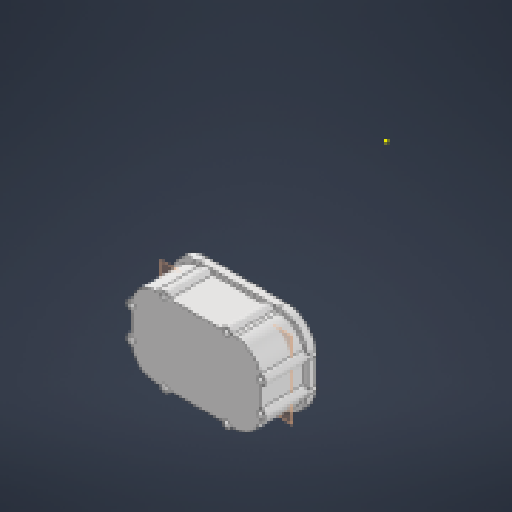
# Autodesk Inventor part: front_main_body
Saved by Autodesk Inventor 2024 (Build 280153000, 153)
## iProperties
Created: 2026-08-19
Part Number: front_main_body
Material: Generic
Document SubType Name: Modeling
Designer: schar
Density: 1 g/cm^3
Appearance: Default
Author: schar
Autodesk Inventor part; units mm, degrees
ref_plane "YZ Plane" through (0, 0, 0) normal (1, 0, 0) x (0, 1, 0)
ref_plane "XZ Plane" through (0, 0, 0) normal (0, 1, 0) x (-1, 0, 0)
ref_plane "XY Plane" through (0, 0, 0) normal (0, 0, 1) x (1, 0, 0)
ref_plane "Work Plane1" through (0, 0, 0) normal (0, 0, 1) x (1, 0, 0)
sketch "Sketch1" plane through (0, 0, 0) normal (0, 0, 1) x (1, 0, 0)
  circle A0 centre (-97.4, -116.425) radius 0.5 projected
  circle A1 centre (-82.2, -105.3) radius 1.6 projected
  circle A2 centre (-57.8, -105.3) radius 1.6 projected
  circle A3 centre (-49.4, -113.69) radius 0.5 projected
  circle A4 centre (-49.4, -116.23) radius 0.5 projected
  circle A5 centre (-97.4, -118.965) radius 0.5 projected
  circle A6 centre (-49.4, -118.77) radius 0.5 projected
  circle A7 centre (-49.4, -121.31) radius 0.5 projected
  circle A8 centre (-82.2, -129.7) radius 1.6 projected
  circle A9 centre (-57.8, -129.7) radius 1.6 projected
  line L0 (-100, -110) -> (-100, -125) projected
  arc A10 (-100, -125) -> (-90, -135) centre (-90, -125) ccw projected
  line L1 (-90, -135) -> (-50, -135) projected
  arc A11 (-50, -135) -> (-40, -125) centre (-50, -125) ccw projected
  line L2 (-40, -125) -> (-40, -110) projected
  arc A12 (-40, -110) -> (-50, -100) centre (-50, -110) ccw projected
  line L3 (-50, -100) -> (-90, -100) projected
  arc A13 (-90, -100) -> (-100, -110) centre (-90, -110) ccw projected
  circle A14 centre (-82.2, -105.3) radius 1.6
  circle A15 centre (-82.2, -105.3) radius 2.5
  circle A16 centre (-57.8, -105.3) radius 1.6
  circle A17 centre (-57.8, -105.3) radius 2.5
  circle A18 centre (-57.8, -129.7) radius 1.6
  circle A19 centre (-57.8, -129.7) radius 2.5
  circle A20 centre (-82.2, -129.7) radius 1.6
  circle A21 centre (-82.2, -129.7) radius 2.5
  line L4 (-90, -97.5) -> (-50, -97.5)
  arc A22 (-37.5, -110) -> (-50, -97.5) centre (-50, -110) ccw
  line L5 (-37.5, -110) -> (-37.5, -125)
  arc A23 (-50, -137.5) -> (-37.5, -125) centre (-50, -125) ccw
  line L6 (-50, -137.5) -> (-90, -137.5)
  arc A24 (-102.5, -125) -> (-90, -137.5) centre (-90, -125) ccw
  line L7 (-102.5, -125) -> (-102.5, -110)
  arc A25 (-90, -97.5) -> (-102.5, -110) centre (-90, -110) ccw
  point P0 (0, 0)
  dimension "d0" = 5
  dimension "d1" = 5
  dimension "d2" = 5
  dimension "d3" = 5
  dimension "d4" = 2.5
  constraints: 12 centre point, 8 coincident, 8 end point, 8 point on circle, 4 concentric, 7 other
  measures "d0" diameter of A15
  measures "d1" diameter of A17
  measures "d2" diameter of A19
  measures "d3" diameter of A21
  measures "d4" distance between parallel lines of L3 L4
extrude "Extrusion1" add sketch "Sketch1" along normal blind 13 contours A15 | A17 | A19 | A21 | L4 A22 L5 A23 L6 A24 L7 A25
sketch "Sketch2" plane through (0, 0, 13) normal (0, 0, 1) x (1, 0, 0)
  line L0 (-50, -97.5) -> (-90, -97.5) projected
  arc A0 (-37.5, -110) -> (-50, -97.5) centre (-50, -110) ccw projected
  line L1 (-37.5, -125) -> (-37.5, -110) projected
  arc A1 (-50, -137.5) -> (-37.5, -125) centre (-50, -125) ccw projected
  line L2 (-90, -137.5) -> (-50, -137.5) projected
  arc A2 (-102.5, -125) -> (-90, -137.5) centre (-90, -125) ccw projected
  line L3 (-102.5, -110) -> (-102.5, -125) projected
  arc A3 (-90, -97.5) -> (-102.5, -110) centre (-90, -110) ccw projected
  point P0 (0, 0)
extrude "Extrusion2" add sketch "Sketch2" along normal blind 2.5
sketch "Sketch3" plane through (0, 0, 0) normal (0, 0, -1) x (-1, 0, 0)
  line L0 (90, -137.5) -> (50, -137.5) projected
  arc A0 (90, -137.5) -> (102.5, -125) centre (90, -125) ccw projected
  line L1 (102.5, -110) -> (102.5, -125) projected
  arc A1 (102.5, -110) -> (90, -97.5) centre (90, -110) ccw projected
  line L2 (50, -97.5) -> (90, -97.5) projected
  arc A2 (50, -97.5) -> (37.5, -110) centre (50, -110) ccw projected
  line L3 (37.5, -125) -> (37.5, -110) projected
  arc A3 (37.5, -125) -> (50, -137.5) centre (50, -125) ccw projected
  arc A4 (100, -110) -> (90, -100) centre (90, -110) ccw projected
  line L4 (100, -125) -> (100, -110) projected
  arc A5 (90, -135) -> (100, -125) centre (90, -125) ccw projected
  line L5 (50, -135) -> (90, -135) projected
  arc A6 (40, -125) -> (50, -135) centre (50, -125) ccw projected
  line L6 (40, -110) -> (40, -125) projected
  arc A7 (50, -100) -> (40, -110) centre (50, -110) ccw projected
  line L7 (90, -100) -> (50, -100) projected
  point P0 (0, 0)
extrude "Extrusion3" add sketch "Sketch3" along normal blind 10
sketch "Sketch4" plane through (-82.2, -129.7, 13) normal (0, 0, -1) x (-1, 0, 0)
  circle A0 centre (0, 0) radius 1.6 projected
  circle A1 centre (0, 24.4) radius 1.6 projected
  circle A2 centre (-24.4, 24.4) radius 1.6 projected
  circle A3 centre (-24.4, 0) radius 1.6 projected
  circle A4 centre (0, 0) radius 1.5
  circle A5 centre (-24.4, 0) radius 1.5
  circle A6 centre (-24.4, 24.4) radius 1.5
  circle A7 centre (0, 24.4) radius 1.5
  point P0 (-82.2, 129.7)
  dimension "d11" = 3
  dimension "d12" = 3
  dimension "d13" = 3
  dimension "d14" = 3
  constraints: 4 centre point, 4 coincident
  measures "d11" diameter of A4
  measures "d12" diameter of A5
  measures "d13" diameter of A6
  measures "d14" diameter of A7
extrude "Extrusion4" add sketch "Sketch4" along normal up to surface (13 mm away)
sketch "Sketch5" plane through (0, 0, -10) normal (0, 0, -1) x (-1, 0, 0)
  line L0 (100, -125) -> (100, -110) projected
  arc A0 (100, -110) -> (90, -100) centre (90, -110) ccw projected
  line L1 (50, -100) -> (90, -100) projected
  arc A1 (50, -100) -> (40, -110) centre (50, -110) ccw projected
  line L2 (40, -125) -> (40, -110) projected
  arc A2 (40, -125) -> (50, -135) centre (50, -125) ccw projected
  line L3 (90, -135) -> (50, -135) projected
  arc A3 (90, -135) -> (100, -125) centre (90, -125) ccw projected
  circle A4 centre (57.8, -129.7) radius 1.6 projected
  circle A5 centre (82.2, -129.7) radius 1.6 projected
  circle A6 centre (49.4, -121.31) radius 0.5 projected
  circle A7 centre (49.4, -118.77) radius 0.5 projected
  circle A8 centre (97.4, -118.965) radius 0.5 projected
  circle A9 centre (49.4, -116.23) radius 0.5 projected
  circle A10 centre (49.4, -113.69) radius 0.5 projected
  circle A11 centre (57.8, -105.3) radius 1.6 projected
  circle A12 centre (82.2, -105.3) radius 1.6 projected
  circle A13 centre (97.4, -116.425) radius 0.5 projected
  arc A14 (100.2, -110) -> (90, -99.8) centre (90, -110) ccw
  line L4 (100.2, -110) -> (100.2, -125)
  arc A15 (90, -135.2) -> (100.2, -125) centre (90, -125) ccw
  line L5 (90, -135.2) -> (50, -135.2)
  arc A16 (39.8, -125) -> (50, -135.2) centre (50, -125) ccw
  line L6 (39.8, -125) -> (39.8, -110)
  arc A17 (50, -99.8) -> (39.8, -110) centre (50, -110) ccw
  line L7 (50, -99.8) -> (90, -99.8)
  point P0 (0, 0)
  dimension "d17" = 0.2
  constraints: 8 end point, 8 point on circle, 4 centre point, 7 other
  measures "d17" distance between parallel lines of L1 L7
extrude "Extrusion5" cut sketch "Sketch5" against normal up to surface (23 mm away) contours L4 A15 L5 A16 L6 A17 L7 A14
sketch "Sketch6" plane through (0, 0, -10) normal (0, 0, -1) x (-1, 0, 0)
  point P0 (0, 0)
sketch "Sketch8" plane through (0, 0, -10) normal (0, 0, -1) x (-1, 0, 0)
  line L0 (90, -99.8) -> (50, -99.8) projected
  line L1 (50, -99.8) -> (54.5, -99.8)
  line L2 (54.5, -99.8) -> (54.5, -97.8)
  circle A0 centre (54.5, -97.8) radius 1.5
  circle A1 centre (54.5, -97.8) radius 2.5
  line L3 (50, -99.8) -> (90, -99.8)
  line L4 (90, -135.2) -> (50, -135.2) projected
  line L5 (50, -135.2) -> (90, -135.2)
  line L6 (90, -135.2) -> (70, -135.2)
  line L7 (50, -99.8) -> (90, -99.8) projected
  line L8 (70, -99.8) -> (70, -135.2)
  circle A2 centre (85.5, -97.8) radius 1.5
  circle A3 centre (85.5, -97.8) radius 2.5
  line L9 (70, -117.5) -> (100.2, -117.5)
  line L10 (100.2, -110) -> (100.2, -125) projected
  circle A4 centre (54.5, -137.2) radius 1.5
  circle A5 centre (54.5, -137.2) radius 2.5
  circle A6 centre (85.5, -137.2) radius 2.5
  circle A7 centre (85.5, -137.2) radius 1.5
  point P0 (0, 0)
  point P1 (53, -135.2)
  point P2 (56, -135.2)
  point P3 (84, -135.2)
  point P4 (87, -135.2)
  point P5 (87, -99.8)
  point P6 (84, -99.8)
  point P7 (56, -99.8)
  point P8 (53, -99.8)
  dimension "d37" = 4.5
  dimension "d38" = 2
  dimension "d39" = 3
  dimension "d40" = 5
  constraints: 14 end point, 8 centre point, 6 symmetric about line, 5 coincident, 4 midpoint, 2 perpendicular, 1 collinear, 1 horizontal, 1 point on line, 6 other
  measures "d37" distance of L0.end L1.end
  measures "d38" distance of L1.end L2.end
  measures "d39" diameter of A0
  measures "d40" diameter of A1
extrude "Extrusion6" add sketch "Sketch8" against normal up to surface (25.5 mm away) contours L0 A3 | L0 A1 | A6 L4 | A5 L4 picked at (85.5603, -99.6297) picked at (55.2169, -99.5838) picked at (85.5603, -135.3703) picked at (54.5603, -135.3703)
sketch "Sketch9" plane through (0, 0, -10) normal (0, 0, -1) x (-1, 0, 0)
  arc A0 (84.0303, -137.5) -> (86.9697, -137.5) centre (85.5, -137.2) ccw projected
  circle A1 centre (85.5, -137.2) radius 1.5
  arc A2 (53.0303, -137.5) -> (55.9697, -137.5) centre (54.5, -137.2) ccw projected
  line L0 (53.0303, -137.5) -> (55.9697, -137.5) projected
  circle A3 centre (54.5, -137.2) radius 1.5
  arc A4 (55.9697, -97.5) -> (53.0303, -97.5) centre (54.5, -97.8) ccw projected
  circle A5 centre (54.5, -97.8) radius 1.5
  arc A6 (86.9697, -97.5) -> (84.0303, -97.5) centre (85.5, -97.8) ccw projected
  circle A7 centre (85.5, -97.8) radius 1.5
  point P0 (0, 0)
  point P1 (86.9697, -97.5)
  constraints: 4 coincident, 2 centre point, 6 other
extrude "Extrusion7" cut sketch "Sketch9" against normal up to surface (25.5 mm away)
sketch "Sketch10" plane through (0, 0, -10) normal (0, 0, -1) x (-1, 0, 0)
  line L0 (37.5, -125) -> (37.5, -110) projected
  circle A0 centre (37.5, -110) radius 1.5
  circle A1 centre (37.5, -125) radius 1.5
  arc A2 (90, -137.5) -> (102.5, -125) centre (90, -125) ccw projected
  circle A3 centre (102.5, -125) radius 1.5
  arc A4 (102.5, -110) -> (90, -97.5) centre (90, -110) ccw projected
  circle A5 centre (102.5, -110) radius 1.5
  circle A6 centre (102.5, -110) radius 2.5
  circle A7 centre (102.5, -125) radius 2.5
  circle A8 centre (37.5, -125) radius 2.5
  circle A9 centre (37.5, -110) radius 2.5
  point P0 (0, 0)
  dimension "d45" = 3
  dimension "d46" = 3
  dimension "d47" = 3
  dimension "d48" = 3
  dimension "d49" = 5
  dimension "d50" = 5
  dimension "d51" = 5
  dimension "d52" = 5
  constraints: 8 centre point, 5 coincident
  measures "d45" diameter of A0
  measures "d46" diameter of A1
  measures "d47" diameter of A3
  measures "d48" diameter of A5
  measures "d49" diameter of A6
  measures "d50" diameter of A7
  measures "d51" diameter of A8
  measures "d52" diameter of A9
extrude "Extrusion8" add sketch "Sketch10" against normal up to surface (25.5 mm away)
sketch "Sketch11" plane through (0, 0, -10) normal (0, 0, -1) x (-1, 0, 0)
  arc A0 (37.59, -108.5027) -> (37.5, -111.5) centre (37.5, -110) ccw projected
  circle A1 centre (37.5, -110) radius 1.5
  arc A2 (37.5, -125) -> (37.59, -126.4973) centre (50, -125) ccw projected
  circle A3 centre (37.5, -125) radius 1.5
  arc A4 (102.41, -126.4973) -> (102.5, -125) centre (90, -125) ccw projected
  circle A5 centre (102.5, -125) radius 1.5
  line L0 (102.5, -111.5) -> (102.5, -110) projected
  circle A6 centre (102.5, -110) radius 1.5
  point P0 (0, 0)
  constraints: 2 coincident, 1 centre point, 1 vertical alignment, 8 other
extrude "Extrusion9" cut sketch "Sketch11" against normal up to surface (25.5 mm away)
sketch "Sketch12" plane through (0, 0, -10) normal (0, 0, -1) x (-1, 0, 0)
  arc A0 (50, -99.8) -> (39.8384, -109.1158) centre (50, -110) ccw projected
  arc A1 (39.8, -110.9798) -> (39.8384, -109.1158) centre (37.5, -110) ccw projected
  line L0 (39.8, -124.0202) -> (39.8, -110.9798) projected
  arc A2 (39.8384, -125.8842) -> (50, -135.2) centre (50, -125) ccw projected
  arc A3 (39.8384, -125.8842) -> (39.8, -124.0202) centre (37.5, -125) ccw projected
  line L1 (90, -135.2) -> (50, -135.2) projected
  arc A4 (90, -135.2) -> (100.1616, -125.8842) centre (90, -125) ccw projected
  line L2 (100.2, -110.9798) -> (100.2, -124.0202) projected
  arc A5 (100.2, -124.0202) -> (100.1616, -125.8842) centre (102.5, -125) ccw projected
  arc A6 (100.1616, -109.1158) -> (90, -99.8) centre (90, -110) ccw projected
  arc A7 (100.1616, -109.1158) -> (100.2, -110.9798) centre (102.5, -110) ccw projected
  line L3 (50, -99.8) -> (90, -99.8) projected
  line L4 (39.8384, -109.1158) -> (39.8, -110.9798)
  line L5 (39.8, -110.9798) -> (39.8384, -109.1158)
  line L6 (39.8, -124.0202) -> (39.8384, -125.8842)
  line L7 (100.2, -124.0202) -> (100.1616, -125.8842)
  line L8 (100.1616, -109.1158) -> (100.2, -110.9798)
  point P0 (0, 0)
  constraints: 10 end point, 2 equal length
extrude "Extrusion10" cut sketch "Sketch12" against normal up to surface (23 mm away) contours A1 L4 | L8 A7 | A3 L6 | L7 A5
sketch "Sketch13" plane through (0, 0, -10) normal (0, 0, -1) x (-1, 0, 0)
  arc A0 (50, -97.5) -> (37.75, -107.5125) centre (50, -110) ccw projected
  line L0 (52.0181, -97.5) -> (50, -97.5) projected
  arc A1 (56.9819, -97.5) -> (52.0181, -97.5) centre (54.5, -97.8) ccw projected
  line L1 (83.0181, -97.5) -> (56.9819, -97.5) projected
  arc A2 (87.9819, -97.5) -> (83.0181, -97.5) centre (85.5, -97.8) ccw projected
  arc A3 (102.25, -107.5125) -> (90, -97.5) centre (90, -110) ccw projected
  line L2 (90, -97.5) -> (87.9819, -97.5) projected
  arc A4 (102.5, -112.5) -> (102.25, -107.5125) centre (102.5, -110) ccw projected
  line L3 (102.5, -122.5) -> (102.5, -112.5) projected
  arc A5 (102.25, -127.4875) -> (102.5, -122.5) centre (102.5, -125) ccw projected
  arc A6 (90, -137.5) -> (102.25, -127.4875) centre (90, -125) ccw projected
  line L4 (87.9819, -137.5) -> (90, -137.5) projected
  arc A7 (83.0181, -137.5) -> (87.9819, -137.5) centre (85.5, -137.2) ccw projected
  line L5 (56.9819, -137.5) -> (83.0181, -137.5) projected
  arc A8 (52.0181, -137.5) -> (56.9819, -137.5) centre (54.5, -137.2) ccw projected
  arc A9 (37.75, -127.4875) -> (50, -137.5) centre (50, -125) ccw projected
  line L6 (50, -137.5) -> (52.0181, -137.5) projected
  arc A10 (37.5, -122.5) -> (37.75, -127.4875) centre (37.5, -125) ccw projected
  line L7 (37.5, -112.5) -> (37.5, -122.5) projected
  arc A11 (37.75, -107.5125) -> (37.5, -112.5) centre (37.5, -110) ccw projected
  circle A12 centre (57.8, -129.7) radius 2.5 projected
  circle A13 centre (82.2, -129.7) radius 2.5 projected
  circle A14 centre (57.8, -105.3) radius 2.5 projected
  circle A15 centre (82.2, -105.3) radius 2.5 projected
  line L8 (100.2, -124.0202) -> (100.2, -110.9798) projected
  line L9 (100.2, -110.9798) -> (100.1616, -109.1158) projected
  arc A16 (100.1616, -109.1158) -> (90, -99.8) centre (90, -110) ccw projected
  line L10 (90, -99.8) -> (50, -99.8) projected
  arc A17 (50, -99.8) -> (39.8384, -109.1158) centre (50, -110) ccw projected
  line L11 (39.8384, -109.1158) -> (39.8, -110.9798) projected
  line L12 (39.8, -110.9798) -> (39.8, -124.0202) projected
  line L13 (39.8, -124.0202) -> (39.8384, -125.8842) projected
  arc A18 (39.8384, -125.8842) -> (50, -135.2) centre (50, -125) ccw projected
  line L14 (50, -135.2) -> (90, -135.2) projected
  arc A19 (90, -135.2) -> (100.1616, -125.8842) centre (90, -125) ccw projected
  line L15 (100.1616, -125.8842) -> (100.2, -124.0202) projected
  line L16 (50, -95.2968) -> (90, -95.2968)
  arc A20 (104.6611, -108.8875) -> (90, -95.2968) centre (90, -110) ccw
  line L17 (104.6611, -108.8875) -> (104.7032, -110.9334)
  line L18 (104.7032, -110.9334) -> (104.7032, -124.0666)
  line L19 (104.7032, -124.0666) -> (104.6611, -126.1125)
  arc A21 (90, -139.7032) -> (104.6611, -126.1125) centre (90, -125) ccw
  line L20 (90, -139.7032) -> (50, -139.7032)
  arc A22 (35.3389, -126.1125) -> (50, -139.7032) centre (50, -125) ccw
  line L21 (35.3389, -126.1125) -> (35.2968, -124.0666)
  line L22 (35.2968, -124.0666) -> (35.2968, -110.9334)
  line L23 (35.2968, -110.9334) -> (35.3389, -108.8875)
  arc A23 (50, -95.2968) -> (35.3389, -108.8875) centre (50, -110) ccw
  point P0 (0, 0)
  point P1 (35.2968, -111.1815)
  point P2 (35.2968, -123.8185)
  point P3 (35.3526, -126.2801)
  point P4 (104.6474, -126.2801)
  point P5 (104.7032, -123.8185)
  point P6 (104.7032, -111.1815)
  point P7 (104.6474, -108.7199)
  point P8 (35.3526, -108.7199)
  constraints: 16 end point, 8 point on circle, 4 centre point, 11 other
extrude "Extrusion11" add sketch "Sketch13" against normal blind 4 contours A0 A11 A23 L16 A20 A4 A3 L2 A2 L1 A1 L0 | A11 L7 A10 L22 | A10 A9 L6 A8 L5 A7 L4 A6 A5 A21 L20 A22 | L18 A5 L3 A4
sketch "Sketch14" plane through (0, 0, -10) normal (0, 0, -1) x (-1, 0, 0)
  line L0 (90, -135.2) -> (50, -135.2) projected
  arc A0 (39.8384, -125.8842) -> (50, -135.2) centre (50, -125) ccw projected
  circle A1 centre (57.8, -129.7) radius 2.5 projected
  circle A2 centre (82.2, -129.7) radius 2.5 projected
  circle A3 centre (57.8, -105.3) radius 2.5 projected
  circle A4 centre (82.2, -105.3) radius 2.5 projected
  line L1 (100.2, -124.0202) -> (100.2, -110.9798) projected
  line L2 (100.2, -110.9798) -> (100.1616, -109.1158) projected
  arc A5 (100.1616, -109.1158) -> (90, -99.8) centre (90, -110) ccw projected
  line L3 (90, -99.8) -> (50, -99.8) projected
  arc A6 (50, -99.8) -> (39.8384, -109.1158) centre (50, -110) ccw projected
  line L4 (39.8384, -109.1158) -> (39.8, -110.9798) projected
  line L5 (39.8, -110.9798) -> (39.8, -124.0202) projected
  line L6 (39.8, -124.0202) -> (39.8384, -125.8842) projected
  arc A7 (39.8384, -125.8842) -> (50, -135.2) centre (50, -125) ccw projected
  line L7 (50, -135.2) -> (90, -135.2) projected
  arc A8 (90, -135.2) -> (100.1616, -125.8842) centre (90, -125) ccw projected
  line L8 (100.1616, -125.8842) -> (100.2, -124.0202) projected
  line L9 (50, -97.8) -> (90, -97.8)
  arc A9 (102.1599, -109.0113) -> (90, -97.8) centre (90, -110) ccw
  line L10 (102.1599, -109.0113) -> (102.2, -110.9592)
  line L11 (102.2, -110.9592) -> (102.2, -124.0408)
  line L12 (102.2, -124.0408) -> (102.1599, -125.9887)
  arc A10 (90, -137.2) -> (102.1599, -125.9887) centre (90, -125) ccw
  line L13 (90, -137.2) -> (50, -137.2)
  arc A11 (37.8401, -125.9887) -> (50, -137.2) centre (50, -125) ccw
  line L14 (37.8401, -125.9887) -> (37.8, -124.0408)
  line L15 (37.8, -124.0408) -> (37.8, -110.9592)
  line L16 (37.8, -110.9592) -> (37.8401, -109.0113)
  arc A12 (50, -97.8) -> (37.8401, -109.0113) centre (50, -110) ccw
  line L17 (90, -97.3) -> (50, -97.3)
  arc A13 (50, -97.3) -> (37.3405, -108.986) centre (50, -110) ccw
  line L18 (37.3405, -108.986) -> (37.3, -110.954)
  line L19 (37.3, -110.954) -> (37.3, -124.046)
  line L20 (37.3, -124.046) -> (37.3405, -126.014)
  arc A14 (37.3405, -126.014) -> (50, -137.7) centre (50, -125) ccw
  line L21 (50, -137.7) -> (90, -137.7)
  arc A15 (90, -137.7) -> (102.6595, -126.014) centre (90, -125) ccw
  line L22 (102.6595, -126.014) -> (102.7, -124.046)
  line L23 (102.7, -124.046) -> (102.7, -110.954)
  line L24 (102.7, -110.954) -> (102.6595, -108.986)
  arc A16 (102.6595, -108.986) -> (90, -97.3) centre (90, -110) ccw
  line L25 (90, -98.3) -> (50, -98.3)
  arc A17 (50, -98.3) -> (38.3397, -109.0369) centre (50, -110) ccw
  line L26 (38.3397, -109.0369) -> (38.3, -110.9643)
  line L27 (38.3, -110.9643) -> (38.3, -124.0357)
  line L28 (38.3, -124.0357) -> (38.3397, -125.9631)
  arc A18 (38.3397, -125.9631) -> (50, -136.7) centre (50, -125) ccw
  line L29 (50, -136.7) -> (90, -136.7)
  arc A19 (90, -136.7) -> (101.6603, -125.9631) centre (90, -125) ccw
  line L30 (101.6603, -125.9631) -> (101.7, -124.0357)
  line L31 (101.7, -124.0357) -> (101.7, -110.9643)
  line L32 (101.7, -110.9643) -> (101.6603, -109.0369)
  arc A20 (101.6603, -109.0369) -> (90, -98.3) centre (90, -110) ccw
  point P0 (0, 0)
  dimension "d69" = 0.5
  dimension "d70" = 0.5
  constraints: 48 end point, 24 point on circle, 12 centre point, 33 other
  measures "d69" distance between parallel lines of L9 L17
  measures "d70" distance between parallel lines of L9 L25
extrude "Extrusion12" cut sketch "Sketch14" against normal blind 1.5 contours L9 A9 L10 L11 L12 A10 L13 A11 L14 L15 L16 A12 | A16 L24 L23 L22 A15 L21 A14 L20 L19 L18 A13 L17
thread "Thread1" size "M3x0.5" class "6H" standard "ANSI Metric M Profile" length 15.103
thread "Thread2" size "M3x0.5" class "6H" standard "ANSI Metric M Profile" length 15.103
thread "Thread3" size "M3x0.5" class "6H" standard "ANSI Metric M Profile" length 15.103
thread "Thread4" size "M3x0.5" class "6H" standard "ANSI Metric M Profile" length 15.103
sketch "Sketch15" plane through (0, 0, 15.5) normal (0, 0, 1) x (1, 0, 0)
  point P0 (0, 0)
ref_plane "Work Plane2" through (-56.9819, -97.5, 15.5) normal (0, -0.4226183, -0.9063078) x (-1, 0, 0)
ref_plane "Work Plane3" through (-56.9819, -100.4583, 9.1558) normal (0, -0.4226183, -0.9063078) x (-1, 0, 0)
ref_plane "Work Plane4" through (-84.0858, -137.7, 15.5) normal (0, 0.9063078, -0.4226183) x (1, 0, 0)
sketch "Sketch21" plane through (-84.0858, -137.7, 15.5) normal (0, 0.9063078, -0.4226183) x (1, 0, 0)
  line L0 (-1.4142, -3.55) -> (-1.4142, -16.2285) projected
  line L1 (29.5858, -16.2285) -> (29.5858, -3.55) projected
  line L2 (-1.4142, -9.8893) -> (29.5858, -9.8893)
  line L3 (29.5858, -9.8893) -> (29.5858, -7.3893)
  line L4 (29.5858, -7.3893) -> (-1.4142, -7.3893)
  line L5 (-1.4142, -7.3893) -> (-1.4142, -9.8893)
  line L6 (31.5858, -11.8893) -> (-3.4142, -11.8893)
  line L7 (-3.4142, -11.8893) -> (-3.4142, -5.3893)
  line L8 (-3.4142, -5.3893) -> (31.5858, -5.3893)
  line L9 (31.5858, -5.3893) -> (31.5858, -11.8893)
  point P0 (84.0858, -44.1468)
  point P1 (-1.4142, -7.3893)
  point P2 (29.5858, -9.8893)
  dimension "d103" = 2.5
  dimension "d104" = 2
  constraints: 16 end point, 4 parallel, 2 perpendicular, 1 horizontal, 1 midpoint, 1 point on line, 3 other
  measures "d103" distance of L3.end L2.end
  measures "d104" distance between parallel lines of L2 L6
extrude "Extrusion17" add sketch "Sketch21" along normal blind 30 contours L0 L6 L7 L8 | L0 L8 L1 L4 | L2 L1 L6 L0 | L1 L8 L9 L6
sketch "Sketch22" plane through (-84.0858, -137.7, 15.5) normal (0, 0.9063078, -0.4226183) x (1, 0, 0)
  line L0 (-1.4142, -9.8893) -> (-1.4142, -7.3893) projected
  line L1 (-1.4142, -7.3893) -> (29.5858, -7.3893) projected
  line L2 (29.5858, -7.3893) -> (29.5858, -9.8893) projected
  line L3 (29.5858, -9.8893) -> (-1.4142, -9.8893) projected
  point P0 (84.0858, -44.1468)
extrude "Extrusion18" cut sketch "Sketch22" along normal blind 30
sketch "Sketch23" plane through (-84.0858, -110.5108, 2.8215) normal (0, 0.9063078, -0.4226183) x (1, 0, 0)
  point P0 (84.0858, -44.1468)
sketch "Sketch24" plane through (-84.0858, -110.5108, 2.8215) normal (0, 0.9063078, -0.4226183) x (1, 0, 0)
  line L0 (31.5858, -5.3893) -> (-3.4142, -5.3893) projected
  line L1 (31.5858, -11.2308) -> (31.5858, -5.3893) projected
  line L2 (31.5858, -11.2308) -> (28.7423, -11.2308) projected
  line L3 (-3.4142, -5.3893) -> (-3.4142, -11.2308) projected
  line L4 (23.8293, -11.2308) -> (4.3423, -11.2308) projected
  line L5 (27.7121, -11.2308) -> (24.8595, -11.2308) projected
  line L6 (3.3121, -11.2308) -> (0.4595, -11.2308) projected
  line L7 (-0.5707, -11.2308) -> (-3.4142, -11.2308) projected
  ellipse E0 centre (26.2858, -12.3297) end of major axis (26.2858, -18.2452) minor radius 2.5 (27.6608, -7.3893) -> (24.9108, -7.3893) ccw projected
  ellipse E1 centre (26.2858, -12.3297) end of major axis (26.2858, -18.2452) minor radius 2.5 (24.9108, -7.3893) -> (24.0085, -9.8893) ccw projected
  ellipse E2 centre (26.2858, -12.3297) end of major axis (26.2858, -18.2452) minor radius 2.5 (24.0085, -9.8893) -> (23.8293, -11.2308) ccw projected
  ellipse E3 centre (26.2858, -12.3297) end of major axis (26.2858, -18.2452) minor radius 2.5 (28.5631, -9.8893) -> (27.6608, -7.3893) ccw projected
  ellipse E4 centre (26.2858, -12.3297) end of major axis (26.2858, -18.2452) minor radius 2.5 (28.7423, -11.2308) -> (28.5631, -9.8893) ccw projected
  ellipse E5 centre (1.8858, -12.3297) end of major axis (1.8858, -18.2452) minor radius 2.5 (4.3423, -11.2308) -> (4.1631, -9.8893) ccw projected
  ellipse E6 centre (1.8858, -12.3297) end of major axis (1.8858, -18.2452) minor radius 2.5 (4.1631, -9.8893) -> (3.2608, -7.3893) ccw projected
  ellipse E7 centre (1.8858, -12.3297) end of major axis (1.8858, -18.2452) minor radius 2.5 (3.2608, -7.3893) -> (0.5108, -7.3893) ccw projected
  ellipse E8 centre (1.8858, -12.3297) end of major axis (1.8858, -18.2452) minor radius 2.5 (0.5108, -7.3893) -> (-0.3915, -9.8893) ccw projected
  ellipse E9 centre (1.8858, -12.3297) end of major axis (1.8858, -18.2452) minor radius 2.5 (-0.3915, -9.8893) -> (-0.5707, -11.2308) ccw projected
  point P0 (84.0858, -44.1468)
  constraints: 10 other
extrude "Extrusion19" add sketch "Sketch24" along normal blind 5
ref_plane "Work Plane5" through (-80.2777, -103.7016, 5.5927) normal (0, 0.9063078, -0.4226183) x (1, 0, 0)
sketch "Sketch25" plane through (-80.2777, -103.7016, 5.5927) normal (0, 0.9063078, -0.4226183) x (1, 0, 0)
  line L0 (-7.2223, -5.8415) -> (-7.2223, 0) projected
  line L1 (27.7777, 0) -> (27.7777, -5.8415) projected
  line L2 (-7.2223, 0) -> (27.7777, 0)
  line L3 (27.7777, 0) -> (27.7777, -5.8415)
  line L4 (27.7777, -5.8415) -> (-7.2223, -5.8415)
  line L5 (-7.2223, -5.8415) -> (-7.2223, 0)
  point P0 (80.2777, -38.7575)
  point P1 (27.7777, 0)
  point P2 (-7.2223, -5.8415)
  constraints: 8 end point, 2 parallel, 1 horizontal, 1 perpendicular
ref_plane "Work Plane6" through (-80.2777, -103.7016, 5.5927) normal (0, -1, 0) x (1, 0, 0)
extrude "Extrusion20" add sketch "Sketch25" along normal up to surface surface through (-50, -99.8, -10) normal (0, 1, 0)
chamfer "Chamfer1" distance 3 angle 45 1 edges at (-70, -124.9479, 15.5)
chamfer "Chamfer2" distance 5 angle 45 4 edges at (-87.5, -126.4479, 15.5) (-87.5, -117.2578, 15.5) (-52.5, -126.4479, 15.5) (-52.5, -117.2578, 15.5)
chamfer "Chamfer3" distance 5 angle 45 1 edges at (-70, -109.5676, 15.5)
sketch "Sketch27" plane through (-37.5, -122.5, 15.5) normal (1, 0, 0) x (0, 0, -1)
  line L0 (15.5, -2.5) -> (15.5, 12.5) projected
  line L1 (17.01, -2.5) -> (17.01, 12.5) projected
  line L2 (15.5, 5) -> (0, 5)
  line L3 (0, 0) -> (0, 10) projected
  circle A0 centre (7.75, 5) radius 3.175
  point P0 (15.5, 122.5)
  dimension "d122" = 6.35
  constraints: 3 midpoint, 2 end point, 1 centre point
  measures "d122" diameter of A0
extrude "Extrusion21" cut sketch "Sketch27" against normal up to surface (2.3 mm away)
sketch "Sketch28" plane through (-37.5, -122.5, 15.5) normal (1, 0, 0) x (0, 0, -1)
  circle A0 centre (7.75, 5) radius 3.175 projected
  line L0 (7.33, 1.8529) -> (8.17, 1.8529)
  line L1 (0, 0) -> (21.5, 0) projected
  line L2 (7.33, 1.8529) -> (8.17, 1.8529)
  line L3 (8.17, 1.8529) -> (8.17, 2.4129)
  line L4 (8.17, 2.4129) -> (7.33, 2.4129)
  line L5 (7.33, 2.4129) -> (7.33, 1.8529)
  point P0 (15.5, 122.5)
  point P1 (8.17, 1.8529)
  dimension "d125" = 0.84
  dimension "d126" = 0.84
  dimension "d127" = 0.56
  constraints: 10 end point, 3 parallel, 2 point on circle, 1 horizontal, 1 perpendicular
  measures "d125" distance of L0.start L0.end
  measures "d126" distance of L4.end L3.end
  measures "d127" distance of L3.end L2.end
extrude "Extrusion22" add sketch "Sketch28" against normal up to surface (2.3 mm away) contours L0 A0 | L5 L4 L3 L0
sketch "Sketch29" plane through (-102.5, -122.5, 15.5) normal (-1, 0, 0) x (0, 0, 1)
  point P0 (-15.5, 122.5)
sketch "Sketch30" plane through (-102.5, -122.5, 15.5) normal (-1, 0, 0) x (0, 0, 1)
  arc A0 (-7.33, 1.8529) -> (-8.17, 1.8529) centre (-7.75, 5) ccw projected
  circle A1 centre (-7.75, 5) radius 3.5
  point P0 (-15.5, 122.5)
  dimension "d130" = 7
  constraints: 1 centre point, 1 coincident
  measures "d130" diameter of A1
extrude "Extrusion23" cut sketch "Sketch30" against normal blind 10
sketch "Sketch31" plane through (-102.5, -122.5, 15.5) normal (-1, 0, 0) x (0, 0, 1)
  circle A0 centre (-7.75, 5) radius 3.5 projected
  circle A1 centre (-7.75, 5) radius 4.55
  point P0 (-15.5, 122.5)
  dimension "d133" = 9.1
  constraints: 1 centre point, 1 coincident
  measures "d133" diameter of A1
extrude "Extrusion24" add sketch "Sketch31" along normal blind 4
sketch "Sketch32" plane through (-100.2, -124.0202, -10) normal (1, 0, 0) x (0, 0, -1)
  circle A0 centre (-17.75, 6.5202) radius 3.5 projected
  circle A1 centre (-17.75, 6.5202) radius 4.55
  point P0 (-10, 124.0202)
  dimension "d136" = 9.1
  constraints: 1 centre point, 1 coincident
  measures "d136" diameter of A1
extrude "Extrusion25" add sketch "Sketch32" along normal blind 3
chamfer "Chamfer4" distance 2 angle 45 1 edges at (-102.5, -117.5, 3.2)
sketch "Sketch33" plane through (-37.5, -122.5, 15.5) normal (1, 0, 0) x (0, 0, -1)
  point P0 (15.5, 122.5)
sketch "Sketch34" plane through (-37.5, -122.5, 15.5) normal (1, 0, 0) x (0, 0, -1)
  point P0 (15.5, 122.5)
body "Solid1"
